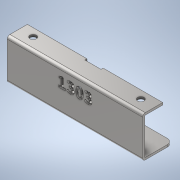
# Autodesk Inventor part: 0 零件
Saved by Autodesk Inventor 2020 (Build 240168000, 168)
## iProperties
Created: 2020-11-03
Part Number: 0 零件
Material: 不鏽鋼
Document SubType Name: Sheet Metal
Designer: p2013
Density: 8 g/cm^3
Appearance: 不鏽鋼 - 疏刷
Sheet Metal Rule: 預設 mm (_M)
Sheet Metal Width: 79.065 mm
Sheet Metal Length: 125.700 mm
Sheet Metal Area: 9938.420 mm^2
Flat Pattern Width: 7.90646 cm
Flat Pattern Length: 12.57 cm
Flat Pattern Area: 99.3842 cm^2
Author: p2013
Autodesk Inventor part; units mm, degrees
ref_plane "YZ Plane" through (0, 0, 0) normal (1, 0, 0) x (0, 1, 0)
ref_plane "XZ Plane" through (0, 0, 0) normal (0, 1, 0) x (-1, 0, 0)
ref_plane "XY Plane" through (0, 0, 0) normal (0, 0, 1) x (1, 0, 0)
sketch "草圖1" plane through (0, 0, 0) normal (0, 0, 1) x (1, 0, 0)
  line L0 (0, -42.8) -> (-53.9141, -42.8) construction
  line L1 (0, -42.8) -> (0, 26.5671) construction
  line L2 (-62.85, 33.5) -> (-7.5, 33.5)
  line L3 (62.85, 33.5) -> (62.85, -42.8)
  line L4 (62.85, -42.8) -> (-62.85, -42.8)
  line L5 (-62.85, -42.8) -> (-62.85, 33.5)
  line L6 (-62.85, 16.5) -> (62.85, 16.5)
  line L7 (-62.85, -16.5) -> (62.85, -16.5)
  line L8 (-62.85, 16.5) -> (62.85, -16.5) construction
  circle A0 centre (-50, 26) radius 3
  line L9 (0, 4) -> (0, 4) construction
  circle A1 centre (50, 26) radius 3
  line L10 (-16.0889, 12) -> (17.4437, 12) construction
  line L11 (17.4437, 12) -> (17.4437, 1.2491) construction
  line L12 (17.4437, 1.2491) -> (-16.0889, 1.2491) construction
  line L13 (-16.0889, 1.2491) -> (-16.0889, 12) construction
  line L14 (7.5, 33.5) -> (0, 33.5) construction
  line L15 (-7.5, 33.5) -> (-7.5, 31.5)
  line L16 (-7.5, 31.5) -> (7.5, 31.5)
  line L17 (7.5, 31.5) -> (7.5, 33.5)
  line L18 (0, 33.5) -> (-7.5, 33.5) construction
  line L19 (7.5, 33.5) -> (62.85, 33.5)
  line L20 (-7.5, 33.5) -> (7.5, 33.5) construction
  line L21 (-15.0397, 1.8313) -> (-15.0397, 3.7608)
  line L22 (-15.0397, 3.7608) -> (-12.9194, 3.7608)
  line L23 (-12.9194, 3.7608) -> (-12.9194, 9.4395)
  line L24 (-12.9194, 9.4395) -> (-14.7609, 9.4395)
  line L25 (-14.7609, 9.4395) -> (-14.7609, 10.9142)
  spline S0 degree 2 poles (-14.7609, 10.9142) (-13.3009, 11.1856) (-12.2884, 11.8313) knots 0 0 0 1 1 1
  line L26 (-12.2884, 11.8313) -> (-11.408, 11.8313)
  line L27 (-11.408, 11.8313) -> (-10.5349, 10.9582)
  line L28 (-10.5349, 10.9582) -> (-10.5349, 3.7608)
  line L29 (-10.5349, 3.7608) -> (-8.7374, 3.7608)
  line L30 (-8.7374, 3.7608) -> (-8.7374, 1.8313)
  line L31 (-8.7374, 1.8313) -> (-15.0397, 1.8313)
  spline S1 degree 2 poles (-4.174, 1.6405) (-6.397, 1.6405) (-7.5929, 3.0418) knots 0 0 0 1 1 1
  line L32 (-7.5929, 3.0418) -> (-6.4924, 4.5385)
  spline S2 degree 2 poles (-6.4924, 4.5385) (-5.4579, 3.5774) (-4.4161, 3.5774) knots 0 0 0 1 1 1
  spline S3 degree 2 poles (-4.4161, 3.5774) (-3.7044, 3.5774) (-3.3009, 3.8709) knots 0 0 0 1 1 1
  spline S4 degree 2 poles (-3.3009, 3.8709) (-2.8827, 4.1643) (-2.8827, 4.7806) knots 0 0 0 1 1 1
  spline S5 degree 2 poles (-2.8827, 4.7806) (-2.8827, 5.4116) (-3.9539, 6.0866) (-4.3427, 6.0205) knots 0 0 0 1 2 2 2
  line L33 (-4.3427, 6.0205) -> (-5.4359, 6.9596)
  line L34 (-5.4359, 6.9596) -> (-5.4359, 7.774)
  spline S6 degree 2 poles (-5.4359, 7.774) (-4.2106, 7.774) (-3.1908, 8.449) (-3.1908, 9.08) knots 0 0 0 1 2 2 2
  spline S7 degree 2 poles (-3.1908, 9.08) (-3.1908, 10.1365) (-4.3354, 10.1365) knots 0 0 0 1 1 1
  spline S8 degree 2 poles (-4.3354, 10.1365) (-5.1791, 10.1365) (-6.1182, 9.3074) knots 0 0 0 1 1 1
  line L35 (-6.1182, 9.3074) -> (-7.3288, 10.7674)
  spline S9 degree 2 poles (-7.3288, 10.7674) (-5.8614, 12) (-2.6406, 12) (-1.7308, 11.281) knots 0 0 0 1 2 2 2
  spline S10 degree 2 poles (-1.7308, 11.281) (-0.8064, 10.5693) (-0.8064, 9.2487) knots 0 0 0 1 1 1
  spline S11 degree 2 poles (-0.8064, 9.2487) (-0.8064, 7.6933) (-2.3985, 6.9817) knots 0 0 0 1 1 1
  spline S12 degree 2 poles (-2.3985, 6.9817) (-1.5254, 6.7175) (-0.4836, 5.4776) (-0.4836, 4.5532) knots 0 0 0 1 2 2 2
  spline S13 degree 2 poles (-0.4836, 4.5532) (-0.4836, 3.2106) (-1.5547, 2.4182) knots 0 0 0 1 1 1
  spline S14 degree 2 poles (-1.5547, 2.4182) (-2.6186, 1.6405) (-4.174, 1.6405) knots 0 0 0 1 1 1
  spline S15 degree 2 poles (6.9266, 2.9978) (5.9728, 1.6405) (2.7299, 1.6405) (0.8077, 4.3551) (0.8077, 9.3881) (2.7299, 12) (5.9728, 12) (7.8803, 9.3734) (7.8803, 4.3551) (6.9266, 2.9978) knots 0 0 0 1 2 3 4 5 6 7 8 8 8
  spline S16 degree 2 poles (3.4049, 4.2304) (3.7497, 3.4967) (4.953, 3.4967) (5.6279, 4.9714) (5.6279, 8.1775) (5.2611, 9.6963) (4.7402, 10.1805) (3.9625, 10.1805) (3.4269, 9.6963) (3.0601, 8.1775) (3.0601, 4.9714) (3.4049, 4.2304) knots 0 0 0 1 2 3 4 5 6 7 8 9 10 10 10
  spline S17 degree 2 poles (12.1723, 1.6405) (9.9493, 1.6405) (8.7534, 3.0418) knots 0 0 0 1 1 1
  line L36 (8.7534, 3.0418) -> (9.8539, 4.5385)
  spline S18 degree 2 poles (9.8539, 4.5385) (10.8884, 3.5774) (11.9302, 3.5774) knots 0 0 0 1 1 1
  spline S19 degree 2 poles (11.9302, 3.5774) (12.6419, 3.5774) (13.0454, 3.8709) knots 0 0 0 1 1 1
  spline S20 degree 2 poles (13.0454, 3.8709) (13.4636, 4.1643) (13.4636, 4.7806) knots 0 0 0 1 1 1
  spline S21 degree 2 poles (13.4636, 4.7806) (13.4636, 5.4116) (12.3924, 6.0866) (12.0036, 6.0205) knots 0 0 0 1 2 2 2
  line L37 (12.0036, 6.0205) -> (10.9104, 6.9596)
  line L38 (10.9104, 6.9596) -> (10.9104, 7.774)
  spline S22 degree 2 poles (10.9104, 7.774) (12.1356, 7.774) (13.1555, 8.449) (13.1555, 9.08) knots 0 0 0 1 2 2 2
  spline S23 degree 2 poles (13.1555, 9.08) (13.1555, 10.1365) (12.0109, 10.1365) knots 0 0 0 1 1 1
  spline S24 degree 2 poles (12.0109, 10.1365) (11.1672, 10.1365) (10.2281, 9.3074) knots 0 0 0 1 1 1
  line L39 (10.2281, 9.3074) -> (9.0175, 10.7674)
  spline S25 degree 2 poles (9.0175, 10.7674) (10.4849, 12) (13.7057, 12) (14.6155, 11.281) knots 0 0 0 1 2 2 2
  spline S26 degree 2 poles (14.6155, 11.281) (15.5399, 10.5693) (15.5399, 9.2487) knots 0 0 0 1 1 1
  spline S27 degree 2 poles (15.5399, 9.2487) (15.5399, 7.6933) (13.9478, 6.9817) knots 0 0 0 1 1 1
  spline S28 degree 2 poles (13.9478, 6.9817) (14.8209, 6.7175) (15.8627, 5.4776) (15.8627, 4.5532) knots 0 0 0 1 2 2 2
  spline S29 degree 2 poles (15.8627, 4.5532) (15.8627, 3.2106) (14.7916, 2.4182) knots 0 0 0 1 1 1
  spline S30 degree 2 poles (14.7916, 2.4182) (13.7277, 1.6405) (12.1723, 1.6405) knots 0 0 0 1 1 1
  point P0 (0, 0)
  point P1 (0, 0)
  point P2 (40.15, 33.5)
  point P3 (28.5517, 33.5)
  dimension "d0" = 125.7
  dimension "d1" = 26.3
  dimension "d2" = 33
  dimension "d3" = 17
  dimension "d11" = 6
  dimension "d15" = 0
  dimension "d18" = 100
  dimension "d36" = 4.5
  dimension "d53" = 7.5
  dimension "d54" = 15
  dimension "d55" = 2
  constraints: 34 end point, 9 point on line, 7 horizontal, 7 parallel, 7 perpendicular, 2 centre point, 2 midpoint, 2 vertical, 1 coincident, 1 symmetric about line, 5 other
  measures "d0" distance between parallel lines of L3 L5
  measures "d1" distance between parallel lines of L7 L4
  measures "d2" distance between parallel lines of L6 L7
  measures "d3" distance between parallel lines of L6 L2
  measures "d11" diameter of A0
  measures "d15" distance of L9.end L9.start
  measures "d18" distance of A1.centre A0.centre
  measures "d36" distance between parallel lines of L6 L10
  measures "d53" distance from line of A1.centre L2
  measures "d54" distance between parallel lines of L17 L15
  measures "d55" distance between parallel lines of L14 L16
extrude "擠出1" add sketch "草圖1" along normal blind 2 contours L2 L15 L16 L17 L19 L3 L6 L5 | L6 L3 L7 L5 | L7 L3 L4 L5 | L21 L22 L23 L24 L25 S0 L26 L27 L28 L29 L30 L31 | S1 L32 S2 S3 S4 S5 L33 L34 S6 S7 S8 L35 S9 S10 S11 S12 S13 S14 | S15 | S16 | S17 L36 S18 S19 S20 S21 L37 L38 S22 S23 S24 L39 S25 S26 S27 S28 S29 S30
extrude "擠出3" cut sketch "草圖1" along normal up to surface (2 mm away) contours L21 L22 L23 L24 L25 S0 L26 L27 L28 L29 L30 L31 | S1 L32 S2 S3 S4 S5 L33 L34 S6 S7 S8 L35 S9 S10 S11 S12 S13 S14 | S15 | S17 L36 S18 S19 S20 S21 L37 L38 S22 S23 S24 L39 S25 S26 S27 S28 S29 S30
sketch "草圖4" plane through (0, 0, 2) normal (0, 0, 1) x (1, 0, 0)
  spline S0 degree 2 poles (6.9266, 2.9978) (5.9728, 1.6405) (2.7299, 1.6405) (0.8077, 4.3551) (0.8077, 9.3881) (2.7299, 12) (5.9728, 12) (7.8803, 9.3734) (7.8803, 4.3551) (6.9266, 2.9978) knots 0 0 0 0.125 0.25 0.375 0.5 0.625 0.75 0.875 1 1 1 projected
  spline S1 degree 2 poles (3.4049, 4.2304) (3.7497, 3.4967) (4.953, 3.4967) (5.6279, 4.9714) (5.6279, 8.1775) (5.2611, 9.6963) (4.7402, 10.1805) (3.9625, 10.1805) (3.4269, 9.6963) (3.0601, 8.1775) (3.0601, 4.9714) (3.4049, 4.2304) knots 0 0 0 0.1 0.2 0.3 0.4 0.5 0.6 0.7 0.8 0.9 1 1 1 projected
  line L0 (0, 10.0218) -> (7.4981, 2.5237)
  line L1 (0.7071, 10.7289) -> (8.2052, 3.2308)
  line L2 (0, 10.0218) -> (0.7071, 10.7289)
  line L3 (7.4981, 2.5237) -> (8.2052, 3.2308)
  line L4 (0, 48.76) -> (0, -58.06) projected
  point P0 (0, 0)
  point P1 (7.4426, 3.9933)
  point P2 (5.607, 5.829)
  point P3 (5.4223, 4.5994)
  point P4 (6.9663, 3.0555)
  point P5 (3.1372, 8.2988)
  point P6 (1.3869, 10.0491)
  point P7 (1.0261, 8.9957)
  point P8 (3.0629, 6.9589)
  dimension "d45" = 45
  dimension "d46" = 1
  dimension "d47" = 7.4981
  dimension "d48" = 10.0218
  constraints: 8 end point, 2 parallel, 1 perpendicular, 1 point on line, 1 vertical alignment, 2 other
  measures "d45" angle of L4 L1
  measures "d46" distance between parallel lines of L0 L1
  measures "d47" horizontal distance of L1.start L1.end
  measures "d48" distance of point (0, 0) L0.start
extrude "擠出4" add sketch "草圖4" against normal up to surface (2 mm away) contours S0 L1 S1 L0 | L0 S1 L1 S0
bend part "折彎零件1" radius 0.5 angle 90 line through (-62.85, 16.5, 0) along (1, 0, 0) centre toward (0, 0, -1) moving side (0, 1, 0) both sides no
bend part "折彎零件2" radius 0.5 angle 90 line through (-62.85, -16.5, 0) along (1, 0, 0) centre toward (0, 0, -1) moving side (0, -1, 0) both sides no
fillet "圓角1" radius 5 2 edges at (62.85, -18, -26.0146) (-62.85, -18, -26.0146)
